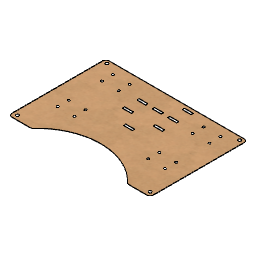
Support_3 (Autodesk Fusion 360 design; units mm, degrees)
Autodesk Fusion 360 part; units mm, degrees
sketch "Esquisse1" plane through (0, 0, 0) normal (0, 1, 0) x (1, 0, 0)
  arc A0 (209.2489, -218.6842) -> (223.8346, -225) centre (223.8346, -205) ccw
  line L0 (-305, 225) -> (305, 225)
  line L1 (215, -225) -> (325, -225)
  line L2 (305, -225) -> (223.8346, -225)
  line L3 (-305, -225) -> (-223.8346, -225)
  line L4 (-325, 225) -> (325, -225) construction
  line L5 (325, 205) -> (325, -205)
  line L6 (-325, -205) -> (-325, 205)
  arc A1 (305, -225) -> (325, -205) centre (305, -205) ccw
  line L7 (-367.4671, -125) -> (350, -125) construction
  arc A2 (-305, 225) -> (-325, 205) centre (-305, 205) ccw
  line L8 (325, 225) -> (-325, -225) construction
  arc A3 (209.2489, -218.6842) -> (-209.2489, -218.6842) centre (0, -415) ccw
  arc A4 (-325, -205) -> (-305, -225) centre (-305, -205) ccw
  arc A5 (-223.8346, -225) -> (-209.2489, -218.6842) centre (-223.8346, -205) ccw
  arc A6 (325, 205) -> (305, 225) centre (305, 205) ccw
  point P0 (-215, -225)
  dimension "d12" = 650
  dimension "d13" = 450
  dimension "d14" = 110
  dimension "d15" = 110
  dimension "d16" = 100
  dimension "d20" = 190
  dimension "d21" = 20
  constraint horizontal L0
  constraint perpendicular L0 L5
  constraint parallel L0 L2
  constraint parallel L5 L6
  constraint coincident origin L4
  constraint coincident origin L8
  constraint coincident P0 L2
  constraint perpendicular L5 L7
  constraint perpendicular L1 L5
  constraint tangent A0 A3
  constraint tangent A0 L2
  constraint coincident L1.end L2
  constraint coincident L1.end L5
  constraint tangent L2 A1
  constraint tangent L5 A1
  constraint equal A0 A1
  constraint coincident L8.start L0
  constraint coincident L8.start L5
  constraint tangent L0 A6
  constraint tangent L5 A6
  constraint equal A0 A6
  constraint coincident L4.start L0
  constraint coincident L4.start L6
  constraint tangent L0 A2
  constraint tangent L6 A2
  constraint equal A0 A2
  constraint coincident L8.end L6
  constraint coincident L8.end L3
  constraint tangent L6 A4
  constraint tangent L3 A4
  constraint equal A0 A4
  constraint coincident P0 L3
  constraint coincident P0 A3
  constraint tangent L3 A5
  constraint tangent A3 A5
  constraint equal A0 A5
  measures "d12" distance of L4.start L8.start
  measures "d13" distance of L4.start L8.end
  measures "d14" distance of P0 L6
  measures "d15" distance of L1.start L5
  measures "d16" distance of L2 L7
  measures "d20" distance of A3.centre L2
  measures "d21" radius of A0
extrude "Extrusion1" add sketch "Esquisse1" along normal blind 1
sketch "Esquisse2" plane through (0, 1, 0) normal (0, 1, 0) x (-1, 0, 0)
  arc A0 (-305, 225) -> (-325, 205) centre (-305, 205) ccw
  line L0 (-325, 205) -> (-325, -205)
  arc A1 (-325, -205) -> (-305, -225) centre (-305, -205) ccw
  line L1 (-305, -225) -> (305, -225)
  arc A2 (305, -225) -> (325, -205) centre (305, -205) ccw
  line L2 (325, -205) -> (325, 205)
  arc A3 (325, 205) -> (305, 225) centre (305, 205) ccw
  line L3 (305, 225) -> (223.8346, 225)
  arc A4 (223.8346, 225) -> (209.2489, 218.6842) centre (223.8346, 205) ccw
  arc A5 (-209.2489, 218.6842) -> (209.2489, 218.6842) centre (0, 415) ccw
  arc A6 (-209.2489, 218.6842) -> (-223.8346, 225) centre (-223.8346, 205) ccw
  line L4 (-223.8346, 225) -> (-305, 225)
  line L5 (-90, -65) -> (-50, -65)
  line L6 (-50, -140) -> (-90, -140)
  line L7 (90, -140) -> (50, -140)
  line L8 (-90, -205) -> (-90, -195)
  line L9 (-50, -75) -> (-90, -75)
  line L10 (-50, -130) -> (-50, -140)
  line L11 (20, -10) -> (-20, -10)
  line L12 (-50, -205) -> (-90, -205)
  line L13 (50, -140) -> (50, -130)
  line L14 (-20, -130) -> (20, -130)
  line L15 (-90, -130) -> (-50, -130)
  line L16 (-50, -195) -> (-50, -205)
  line L17 (50, -65) -> (90, -65)
  line L18 (20, -140) -> (-20, -140)
  line L19 (-90, -75) -> (-90, -65)
  line L20 (-20, -140) -> (-20, -130)
  line L21 (-90, -140) -> (-90, -130)
  line L22 (90, -130) -> (90, -140)
  line L23 (-90, -195) -> (-50, -195)
  line L24 (-20, -10) -> (-20, 0)
  line L25 (90, -65) -> (90, -75)
  line L26 (90, -75) -> (50, -75)
  line L27 (20, 0) -> (20, -10)
  line L28 (50, -75) -> (50, -65)
  line L29 (-50, -65) -> (-50, -75)
  line L30 (20, -130) -> (20, -140)
  line L31 (-20, 0) -> (20, 0)
  line L32 (50, -130) -> (90, -130)
  dimension "d17" = 70
  dimension "d18" = -130
  dimension "d23" = 0
  dimension "d24" = -65
  constraint horizontal L11
  constraint vertical L24
  constraint horizontal L31
  constraint vertical L27
extrude "Extrusion2" cut sketch "Esquisse2" against normal blind 50 contours L5 L9 L19 L29 | L6 L10 L15 L21 | L7 L13 L22 L32 | L8 L12 L16 L23 | L11 L24 L27 L31 | L14 L18 L20 L30 | L17 L25 L26 L28
sketch "Esquisse4" plane through (0, 1, 0) normal (0, 1, 0) x (-1, 0, 0)
  line L0 (90, -65) -> (90, -75)
  line L1 (90, -75) -> (50, -75)
  line L2 (50, -75) -> (50, -65)
  line L3 (50, -65) -> (90, -65)
  line L4 (-50, -205) -> (-90, -205)
  line L5 (-90, -205) -> (-90, -195)
  line L6 (-90, -195) -> (-50, -195)
  line L7 (-50, -195) -> (-50, -205)
  line L8 (90, -140) -> (50, -140)
  line L9 (50, -140) -> (50, -130)
  line L10 (50, -130) -> (90, -130)
  line L11 (90, -130) -> (90, -140)
  line L12 (20, -10) -> (-20, -10)
  line L13 (-20, -10) -> (-20, 0)
  line L14 (-20, 0) -> (20, 0)
  line L15 (20, 0) -> (20, -10)
  line L16 (-50, -130) -> (-50, -140)
  line L17 (-50, -140) -> (-90, -140)
  line L18 (-90, -140) -> (-90, -130)
  line L19 (-90, -130) -> (-50, -130)
  line L20 (-20, -140) -> (-20, -130)
  line L21 (-20, -130) -> (20, -130)
  line L22 (20, -130) -> (20, -140)
  line L23 (20, -140) -> (-20, -140)
  line L24 (-90, -75) -> (-90, -65)
  line L25 (-90, -65) -> (-50, -65)
  line L26 (-50, -65) -> (-50, -75)
  line L27 (-50, -75) -> (-90, -75)
  arc A0 (-305, 225) -> (-325, 205) centre (-305, 205) ccw
  line L28 (-325, 205) -> (-325, -205)
  arc A1 (-325, -205) -> (-305, -225) centre (-305, -205) ccw
  line L29 (-305, -225) -> (305, -225)
  arc A2 (305, -225) -> (325, -205) centre (305, -205) ccw
  line L30 (325, -205) -> (325, 205)
  arc A3 (325, 205) -> (305, 225) centre (305, 205) ccw
  line L31 (305, 225) -> (223.8346, 225)
  arc A4 (223.8346, 225) -> (209.2489, 218.6842) centre (223.8346, 205) ccw
  arc A5 (-209.2489, 218.6842) -> (209.2489, 218.6842) centre (0, 415) ccw
  arc A6 (-209.2489, 218.6842) -> (-223.8346, 225) centre (-223.8346, 205) ccw
  line L32 (-223.8346, 225) -> (-305, 225)
  circle A7 centre (300, -205) radius 6.5
  circle A8 centre (300, 200) radius 6.5
  circle A9 centre (-300, 200) radius 6.5
  circle A10 centre (-300, -205) radius 6.5
  dimension "d43" = 13
  dimension "d46" = 13
  dimension "d49" = 13
  dimension "d52" = 13
  measures "d43" diameter of A7
  measures "d46" diameter of A8
  measures "d49" diameter of A9
  measures "d52" diameter of A10
extrude "Extrusion3" cut sketch "Esquisse4" against normal blind 50 contours A7 | A8 | A9 | A10
sketch "Esquisse5" plane through (0, 1, 0) normal (0, 1, 0) x (-1, 0, 0)
  circle A0 centre (300, 200) radius 6.5
  circle A1 centre (-300, -205) radius 6.5
  circle A2 centre (300, -205) radius 6.5
  circle A3 centre (-300, 200) radius 6.5
  line L0 (90, -65) -> (90, -75)
  line L1 (90, -75) -> (50, -75)
  line L2 (50, -75) -> (50, -65)
  line L3 (50, -65) -> (90, -65)
  line L4 (-50, -205) -> (-90, -205)
  line L5 (-90, -205) -> (-90, -195)
  line L6 (-90, -195) -> (-50, -195)
  line L7 (-50, -195) -> (-50, -205)
  line L8 (90, -140) -> (50, -140)
  line L9 (50, -140) -> (50, -130)
  line L10 (50, -130) -> (90, -130)
  line L11 (90, -130) -> (90, -140)
  line L12 (20, -10) -> (-20, -10)
  line L13 (-20, -10) -> (-20, 0)
  line L14 (-20, 0) -> (20, 0)
  line L15 (20, 0) -> (20, -10)
  line L16 (-50, -130) -> (-50, -140)
  line L17 (-50, -140) -> (-90, -140)
  line L18 (-90, -140) -> (-90, -130)
  line L19 (-90, -130) -> (-50, -130)
  line L20 (-20, -140) -> (-20, -130)
  line L21 (-20, -130) -> (20, -130)
  line L22 (20, -130) -> (20, -140)
  line L23 (20, -140) -> (-20, -140)
  line L24 (-90, -75) -> (-90, -65)
  line L25 (-90, -65) -> (-50, -65)
  line L26 (-50, -65) -> (-50, -75)
  line L27 (-50, -75) -> (-90, -75)
  arc A4 (-305, 225) -> (-325, 205) centre (-305, 205) ccw
  line L28 (-325, 205) -> (-325, -205)
  arc A5 (-325, -205) -> (-305, -225) centre (-305, -205) ccw
  line L29 (-305, -225) -> (305, -225)
  arc A6 (305, -225) -> (325, -205) centre (305, -205) ccw
  line L30 (325, -205) -> (325, 205)
  arc A7 (325, 205) -> (305, 225) centre (305, 205) ccw
  line L31 (305, 225) -> (223.8346, 225)
  arc A8 (223.8346, 225) -> (209.2489, 218.6842) centre (223.8346, 205) ccw
  arc A9 (-209.2489, 218.6842) -> (209.2489, 218.6842) centre (0, 415) ccw
  arc A10 (-209.2489, 218.6842) -> (-223.8346, 225) centre (-223.8346, 205) ccw
  line L32 (-223.8346, 225) -> (-305, 225)
  circle A11 centre (167, 75) radius 5
  circle A12 centre (243, 25) radius 5
  circle A13 centre (167, -175) radius 5
  circle A14 centre (243, -125) radius 5
  circle A15 centre (167, 25) radius 5
  circle A16 centre (243, -175) radius 5
  circle A17 centre (167, -125) radius 5
  circle A18 centre (243, 75) radius 5
  circle A19 centre (-243, 75) radius 5
  circle A20 centre (-243, -175) radius 5
  circle A21 centre (-243, 25) radius 5
  circle A22 centre (-167, 25) radius 5
  circle A23 centre (-167, -175) radius 5
  circle A24 centre (-167, -125) radius 5
  circle A25 centre (-243, -125) radius 5
  circle A26 centre (-167, 75) radius 5
  dimension "d60" = 10
  measures "d60" diameter of A20
extrude "Extrusion4" cut sketch "Esquisse5" against normal blind 75 contours A11 | A12 | A13 | A14 | A15 | A16 | A17 | A18 | A19 | A20 | A21 | A22 | A23 | A24 | A25 | A26
sketch "Esquisse6" plane through (0, 1, 0) normal (0, 1, 0) x (-1, 0, 0)
  circle A0 centre (243, 25) radius 5
  circle A1 centre (-243, 25) radius 5
  circle A2 centre (-243, -175) radius 5
  circle A3 centre (243, -125) radius 5
  circle A4 centre (167, -175) radius 5
  circle A5 centre (-243, -125) radius 5
  circle A6 centre (-243, 75) radius 5
  circle A7 centre (243, 75) radius 5
  circle A8 centre (167, 25) radius 5
  circle A9 centre (-167, 25) radius 5
  circle A10 centre (-167, -175) radius 5
  circle A11 centre (243, -175) radius 5
  circle A12 centre (167, -125) radius 5
  circle A13 centre (-167, -125) radius 5
  circle A14 centre (-167, 75) radius 5
  circle A15 centre (167, 75) radius 5
  circle A16 centre (300, 200) radius 6.5
  circle A17 centre (-300, -205) radius 6.5
  circle A18 centre (300, -205) radius 6.5
  circle A19 centre (-300, 200) radius 6.5
  line L0 (90, -65) -> (90, -75)
  line L1 (90, -75) -> (50, -75)
  line L2 (50, -75) -> (50, -65)
  line L3 (50, -65) -> (90, -65)
  line L4 (-50, -205) -> (-90, -205)
  line L5 (-90, -205) -> (-90, -195)
  line L6 (-90, -195) -> (-50, -195)
  line L7 (-50, -195) -> (-50, -205)
  line L8 (90, -140) -> (50, -140)
  line L9 (50, -140) -> (50, -130)
  line L10 (50, -130) -> (90, -130)
  line L11 (90, -130) -> (90, -140)
  line L12 (20, -10) -> (-20, -10)
  line L13 (-20, -10) -> (-20, 0)
  line L14 (-20, 0) -> (20, 0)
  line L15 (20, 0) -> (20, -10)
  line L16 (-50, -130) -> (-50, -140)
  line L17 (-50, -140) -> (-90, -140)
  line L18 (-90, -140) -> (-90, -130)
  line L19 (-90, -130) -> (-50, -130)
  line L20 (-20, -140) -> (-20, -130)
  line L21 (-20, -130) -> (20, -130)
  line L22 (20, -130) -> (20, -140)
  line L23 (20, -140) -> (-20, -140)
  line L24 (-90, -75) -> (-90, -65)
  line L25 (-90, -65) -> (-50, -65)
  line L26 (-50, -65) -> (-50, -75)
  line L27 (-50, -75) -> (-90, -75)
  arc A20 (-305, 225) -> (-325, 205) centre (-305, 205) ccw
  line L28 (-325, 205) -> (-325, -205)
  arc A21 (-325, -205) -> (-305, -225) centre (-305, -205) ccw
  line L29 (-305, -225) -> (305, -225)
  arc A22 (305, -225) -> (325, -205) centre (305, -205) ccw
  line L30 (325, -205) -> (325, 205)
  arc A23 (325, 205) -> (305, 225) centre (305, 205) ccw
  line L31 (305, 225) -> (223.8346, 225)
  arc A24 (223.8346, 225) -> (209.2489, 218.6842) centre (223.8346, 205) ccw
  arc A25 (-209.2489, 218.6842) -> (209.2489, 218.6842) centre (0, 415) ccw
  arc A26 (-209.2489, 218.6842) -> (-223.8346, 225) centre (-223.8346, 205) ccw
  line L32 (-223.8346, 225) -> (-305, 225)
  line L33 (305, 220) -> (223.8346, 220)
  arc A27 (223.8346, 220) -> (212.8953, 215.2631) centre (223.8346, 205) ccw
  arc A28 (-212.8953, 215.2631) -> (212.8953, 215.2631) centre (0, 415) ccw
  arc A29 (-212.8953, 215.2631) -> (-223.8346, 220) centre (-223.8346, 205) ccw
  line L34 (-223.8346, 220) -> (-305, 220)
  arc A30 (-305, 220) -> (-320, 205) centre (-305, 205) ccw
  line L35 (-320, 205) -> (-320, -205)
  arc A31 (-320, -205) -> (-305, -220) centre (-305, -205) ccw
  line L36 (-305, -220) -> (305, -220)
  arc A32 (305, -220) -> (320, -205) centre (305, -205) ccw
  line L37 (320, -205) -> (320, 205)
  arc A33 (320, 205) -> (305, 220) centre (305, 205) ccw
  dimension "d36" = -5
extrude "Extrusion5" cut sketch "Esquisse6" against normal blind 50 contours A20 L28 A21 L29 A22 L30 A23 L31 A24 A25 A26 L32
sketch "Esquisse7" plane through (0, 1, 0) normal (0, 1, 0) x (-1, 0, 0)
  arc A0 (-212.8953, 215.2631) -> (212.8953, 215.2631) centre (0, 415) ccw
  arc A1 (-212.8953, 215.2631) -> (-223.8346, 220) centre (-223.8346, 205) ccw
  line L0 (-223.8346, 220) -> (-305, 220)
  arc A2 (-305, 220) -> (-320, 205) centre (-305, 205) ccw
  line L1 (-320, 205) -> (-320, -205)
  arc A3 (-320, -205) -> (-305, -220) centre (-305, -205) ccw
  line L2 (-305, -220) -> (305, -220)
  arc A4 (305, -220) -> (320, -205) centre (305, -205) ccw
  line L3 (320, -205) -> (320, 205)
  arc A5 (320, 205) -> (305, 220) centre (305, 205) ccw
  line L4 (305, 220) -> (223.8346, 220)
  arc A6 (223.8346, 220) -> (212.8953, 215.2631) centre (223.8346, 205) ccw
  circle A7 centre (243, 25) radius 5
  circle A8 centre (-243, 25) radius 5
  circle A9 centre (-243, -175) radius 5
  circle A10 centre (243, -125) radius 5
  circle A11 centre (167, -175) radius 5
  circle A12 centre (-243, -125) radius 5
  circle A13 centre (-243, 75) radius 5
  circle A14 centre (243, 75) radius 5
  circle A15 centre (167, 25) radius 5
  circle A16 centre (-167, 25) radius 5
  circle A17 centre (-167, -175) radius 5
  circle A18 centre (243, -175) radius 5
  circle A19 centre (167, -125) radius 5
  circle A20 centre (-167, -125) radius 5
  circle A21 centre (-167, 75) radius 5
  circle A22 centre (167, 75) radius 5
  circle A23 centre (300, 200) radius 6.5
  circle A24 centre (-300, -205) radius 6.5
  circle A25 centre (300, -205) radius 6.5
  circle A26 centre (-300, 200) radius 6.5
  line L5 (90, -65) -> (90, -75)
  line L6 (90, -75) -> (50, -75)
  line L7 (50, -75) -> (50, -65)
  line L8 (50, -65) -> (90, -65)
  line L9 (-50, -205) -> (-90, -205)
  line L10 (-90, -205) -> (-90, -195)
  line L11 (-90, -195) -> (-50, -195)
  line L12 (-50, -195) -> (-50, -205)
  line L13 (90, -140) -> (50, -140)
  line L14 (50, -140) -> (50, -130)
  line L15 (50, -130) -> (90, -130)
  line L16 (90, -130) -> (90, -140)
  line L17 (20, -10) -> (-20, -10)
  line L18 (-20, -10) -> (-20, 0)
  line L19 (-20, 0) -> (20, 0)
  line L20 (20, 0) -> (20, -10)
  line L21 (-50, -130) -> (-50, -140)
  line L22 (-50, -140) -> (-90, -140)
  line L23 (-90, -140) -> (-90, -130)
  line L24 (-90, -130) -> (-50, -130)
  line L25 (-20, -140) -> (-20, -130)
  line L26 (-20, -130) -> (20, -130)
  line L27 (20, -130) -> (20, -140)
  line L28 (20, -140) -> (-20, -140)
  line L29 (-90, -75) -> (-90, -65)
  line L30 (-90, -65) -> (-50, -65)
  line L31 (-50, -65) -> (-50, -75)
  line L32 (-50, -75) -> (-90, -75)
  line L33 (-50, -195) -> (-90, -195)
  line L34 (-90, -195) -> (-90, -155)
  line L35 (-90, -155) -> (-50, -155)
  line L36 (-50, -155) -> (-50, -195)
  line L37 (90, -130) -> (50, -130)
  line L38 (50, -130) -> (50, -90)
  line L39 (50, -90) -> (90, -90)
  line L40 (90, -90) -> (90, -130)
  line L41 (20, -130) -> (-20, -130)
  line L42 (-20, -130) -> (-20, -90)
  line L43 (-20, -90) -> (20, -90)
  line L44 (20, -90) -> (20, -130)
  line L45 (-50, -130) -> (-90, -130)
  line L46 (-90, -130) -> (-90, -90)
  line L47 (-90, -90) -> (-50, -90)
  line L48 (-50, -90) -> (-50, -130)
  line L49 (20, 0) -> (-20, 0)
  line L50 (-20, 0) -> (-20, 40)
  line L51 (-20, 40) -> (20, 40)
  line L52 (20, 40) -> (20, 0)
  line L53 (90, -65) -> (50, -65)
  line L54 (50, -65) -> (50, -25)
  line L55 (50, -25) -> (90, -25)
  line L56 (90, -25) -> (90, -65)
  line L57 (-50, -65) -> (-90, -65)
  line L58 (-90, -65) -> (-90, -25)
  line L59 (-90, -25) -> (-50, -25)
  line L60 (-50, -25) -> (-50, -65)
  line L61 (315, -190) -> (95, -190)
  line L62 (95, -190) -> (95, 120)
  line L63 (95, 120) -> (315, 120)
  line L64 (315, 120) -> (315, -190)
  line L65 (0, -325) -> (0, 200)
  line L66 (-315, 120) -> (-315, -190)
  line L67 (-315, -190) -> (-95, -190)
  line L68 (-95, -190) -> (-95, 120)
  line L69 (-95, 120) -> (-315, 120)
  dimension "d39" = 40
  dimension "d40" = 40
  dimension "d41" = 220
  dimension "d42" = 310
  dimension "d44" = 5
  dimension "d45" = 30
  constraint horizontal L33
  constraint vertical L34
  constraint horizontal L35
  constraint vertical L36
  constraint coincident L11.end L12.start
  constraint horizontal L37
  constraint vertical L38
  constraint horizontal L39
  constraint vertical L40
  constraint coincident L15.end L16.start
  constraint horizontal L41
  constraint vertical L42
  constraint horizontal L43
  constraint vertical L44
  constraint coincident L26.end L27.start
  constraint horizontal L45
  constraint vertical L46
  constraint horizontal L47
  constraint vertical L48
  constraint coincident L21.start L24.end
  constraint horizontal L49
  constraint vertical L50
  constraint horizontal L51
  constraint vertical L52
  constraint coincident L19.end L20.start
  constraint horizontal L53
  constraint vertical L54
  constraint horizontal L55
  constraint vertical L56
  constraint coincident L5.start L8.end
  constraint horizontal L57
  constraint vertical L58
  constraint horizontal L59
  constraint vertical L60
  constraint coincident L30.end L31.start
  constraint horizontal L61
  constraint vertical L62
  constraint horizontal L63
  constraint vertical L64
  constraint perpendicular L51 L65
  constraint symmetric L61.start L65 L66.end
  constraint symmetric L61.end L65 L67.end
  constraint symmetric L62.end L65 L68.end
  constraint symmetric L63.end L65 L66.start
  measures "d39" distance of L34.end L35.end
  measures "d40" distance of L10.end L34.end
  measures "d41" distance of L61.start L61.end
  measures "d42" distance of L61.start L63.end
  measures "d44" distance of L3 L64
  measures "d45" distance of L2 L61
sketch "Esquisse8" plane through (0, 1, 0) normal (0, 1, 0) x (-1, 0, 0)
  arc A0 (-212.8953, 215.2631) -> (212.8953, 215.2631) centre (0, 415) ccw
  arc A1 (-212.8953, 215.2631) -> (-223.8346, 220) centre (-223.8346, 205) ccw
  line L0 (-223.8346, 220) -> (-305, 220)
  arc A2 (-305, 220) -> (-320, 205) centre (-305, 205) ccw
  line L1 (-320, 205) -> (-320, -205)
  arc A3 (-320, -205) -> (-305, -220) centre (-305, -205) ccw
  line L2 (-305, -220) -> (305, -220)
  arc A4 (305, -220) -> (320, -205) centre (305, -205) ccw
  line L3 (320, -205) -> (320, 205)
  arc A5 (320, 205) -> (305, 220) centre (305, 205) ccw
  line L4 (305, 220) -> (223.8346, 220)
  arc A6 (223.8346, 220) -> (212.8953, 215.2631) centre (223.8346, 205) ccw
  circle A7 centre (243, 25) radius 5
  circle A8 centre (-243, 25) radius 5
  circle A9 centre (-243, -175) radius 5
  circle A10 centre (243, -125) radius 5
  circle A11 centre (167, -175) radius 5
  circle A12 centre (-243, -125) radius 5
  circle A13 centre (-243, 75) radius 5
  circle A14 centre (243, 75) radius 5
  circle A15 centre (167, 25) radius 5
  circle A16 centre (-167, 25) radius 5
  circle A17 centre (-167, -175) radius 5
  circle A18 centre (243, -175) radius 5
  circle A19 centre (167, -125) radius 5
  circle A20 centre (-167, -125) radius 5
  circle A21 centre (-167, 75) radius 5
  circle A22 centre (167, 75) radius 5
  circle A23 centre (300, 200) radius 6.5
  circle A24 centre (-300, -205) radius 6.5
  circle A25 centre (300, -205) radius 6.5
  circle A26 centre (-300, 200) radius 6.5
  line L5 (90, -65) -> (90, -75)
  line L6 (90, -75) -> (50, -75)
  line L7 (50, -75) -> (50, -65)
  line L8 (50, -65) -> (90, -65)
  line L9 (-50, -205) -> (-90, -205)
  line L10 (-90, -205) -> (-90, -195)
  line L11 (-90, -195) -> (-50, -195)
  line L12 (-50, -195) -> (-50, -205)
  line L13 (90, -140) -> (50, -140)
  line L14 (50, -140) -> (50, -130)
  line L15 (50, -130) -> (90, -130)
  line L16 (90, -130) -> (90, -140)
  line L17 (20, -10) -> (-20, -10)
  line L18 (-20, -10) -> (-20, 0)
  line L19 (-20, 0) -> (20, 0)
  line L20 (20, 0) -> (20, -10)
  line L21 (-50, -130) -> (-50, -140)
  line L22 (-50, -140) -> (-90, -140)
  line L23 (-90, -140) -> (-90, -130)
  line L24 (-90, -130) -> (-50, -130)
  line L25 (-20, -140) -> (-20, -130)
  line L26 (-20, -130) -> (20, -130)
  line L27 (20, -130) -> (20, -140)
  line L28 (20, -140) -> (-20, -140)
  line L29 (-90, -75) -> (-90, -65)
  line L30 (-90, -65) -> (-50, -65)
  line L31 (-50, -65) -> (-50, -75)
  line L32 (-50, -75) -> (-90, -75)
sketch "Esquisse9" plane through (0, 0, 0) normal (0, -1, 0) x (1, 0, 0)
  arc A0 (-212.8953, 215.2631) -> (212.8953, 215.2631) centre (0, 415) ccw
  arc A1 (-212.8953, 215.2631) -> (-223.8346, 220) centre (-223.8346, 205) ccw
  line L0 (-223.8346, 220) -> (-305, 220)
  arc A2 (-305, 220) -> (-320, 205) centre (-305, 205) ccw
  line L1 (-320, 205) -> (-320, -205)
  arc A3 (-320, -205) -> (-305, -220) centre (-305, -205) ccw
  line L2 (-305, -220) -> (305, -220)
  arc A4 (305, -220) -> (320, -205) centre (305, -205) ccw
  line L3 (320, -205) -> (320, 205)
  arc A5 (320, 205) -> (305, 220) centre (305, 205) ccw
  line L4 (305, 220) -> (223.8346, 220)
  arc A6 (223.8346, 220) -> (212.8953, 215.2631) centre (223.8346, 205) ccw
  circle A7 centre (-243, 25) radius 5
  circle A8 centre (243, 25) radius 5
  circle A9 centre (243, -175) radius 5
  circle A10 centre (-243, -125) radius 5
  circle A11 centre (-167, -175) radius 5
  circle A12 centre (243, -125) radius 5
  circle A13 centre (243, 75) radius 5
  circle A14 centre (-243, 75) radius 5
  circle A15 centre (-167, 25) radius 5
  circle A16 centre (167, 25) radius 5
  circle A17 centre (167, -175) radius 5
  circle A18 centre (-243, -175) radius 5
  circle A19 centre (-167, -125) radius 5
  circle A20 centre (167, -125) radius 5
  circle A21 centre (167, 75) radius 5
  circle A22 centre (-167, 75) radius 5
  circle A23 centre (-300, 200) radius 6.5
  circle A24 centre (300, -205) radius 6.5
  circle A25 centre (-300, -205) radius 6.5
  circle A26 centre (300, 200) radius 6.5
  line L5 (-90, -75) -> (-90, -65)
  line L6 (-90, -65) -> (-50, -65)
  line L7 (-50, -65) -> (-50, -75)
  line L8 (-50, -75) -> (-90, -75)
  line L9 (90, -205) -> (50, -205)
  line L10 (50, -205) -> (50, -195)
  line L11 (50, -195) -> (90, -195)
  line L12 (90, -195) -> (90, -205)
  line L13 (-50, -140) -> (-90, -140)
  line L14 (-90, -140) -> (-90, -130)
  line L15 (-90, -130) -> (-50, -130)
  line L16 (-50, -130) -> (-50, -140)
  line L17 (20, -10) -> (-20, -10)
  line L18 (-20, -10) -> (-20, 0)
  line L19 (-20, 0) -> (20, 0)
  line L20 (20, 0) -> (20, -10)
  line L21 (50, -140) -> (50, -130)
  line L22 (50, -130) -> (90, -130)
  line L23 (90, -130) -> (90, -140)
  line L24 (90, -140) -> (50, -140)
  line L25 (20, -130) -> (20, -140)
  line L26 (20, -140) -> (-20, -140)
  line L27 (-20, -140) -> (-20, -130)
  line L28 (-20, -130) -> (20, -130)
  line L29 (90, -65) -> (90, -75)
  line L30 (90, -75) -> (50, -75)
  line L31 (50, -75) -> (50, -65)
  line L32 (50, -65) -> (90, -65)
  line L33 (-20, 0) -> (20, 0)
  line L34 (20, 0) -> (20, 40)
  line L35 (20, 40) -> (-20, 40)
  line L36 (-20, 40) -> (-20, 0)
  line L37 (-90, -65) -> (-50, -65)
  line L38 (-50, -65) -> (-50, -25)
  line L39 (-50, -25) -> (-90, -25)
  line L40 (-90, -25) -> (-90, -65)
  line L41 (-90, -130) -> (-50, -130)
  line L42 (-50, -130) -> (-50, -90)
  line L43 (-50, -90) -> (-90, -90)
  line L44 (-90, -90) -> (-90, -130)
  line L45 (-20, -130) -> (20, -130)
  line L46 (20, -130) -> (20, -90)
  line L47 (20, -90) -> (-20, -90)
  line L48 (-20, -90) -> (-20, -130)
  line L49 (50, -130) -> (90, -130)
  line L50 (90, -130) -> (90, -90)
  line L51 (90, -90) -> (50, -90)
  line L52 (50, -90) -> (50, -130)
  line L53 (50, -65) -> (90, -65)
  line L54 (90, -65) -> (90, -25)
  line L55 (90, -25) -> (50, -25)
  line L56 (50, -25) -> (50, -65)
  line L57 (50, -195) -> (90, -195)
  line L58 (90, -195) -> (90, -155)
  line L59 (90, -155) -> (50, -155)
  line L60 (50, -155) -> (50, -195)
  dimension "d47" = 40
  dimension "d48" = 40
  dimension "d50" = 40
  dimension "d51" = 40
  dimension "d53" = 40
  dimension "d54" = 40
  dimension "d55" = 40
  constraint horizontal L33
  constraint vertical L34
  constraint horizontal L35
  constraint vertical L36
  constraint coincident L18.end L19.start
  constraint horizontal L37
  constraint vertical L38
  constraint horizontal L39
  constraint vertical L40
  constraint coincident L5.end L6.start
  constraint horizontal L41
  constraint vertical L42
  constraint horizontal L43
  constraint vertical L44
  constraint coincident L14.end L15.start
  constraint horizontal L45
  constraint vertical L46
  constraint horizontal L47
  constraint vertical L48
  constraint coincident L27.end L28.start
  constraint horizontal L49
  constraint vertical L50
  constraint horizontal L51
  constraint vertical L52
  constraint coincident L21.end L22.start
  constraint horizontal L53
  constraint vertical L54
  constraint horizontal L55
  constraint vertical L56
  constraint coincident L31.end L32.start
  constraint horizontal L57
  constraint vertical L58
  constraint horizontal L59
  constraint vertical L60
  constraint coincident L10.end L11.start
  measures "d47" distance of L5.end L39.end
  measures "d48" distance of L18.end L35.end
  measures "d50" distance of L31.end L55.end
  measures "d51" distance of L27.end L47.end
  measures "d53" distance of L14.end L43.end
  measures "d54" distance of L22.end L50.end
  measures "d55" distance of L11.end L58.end
